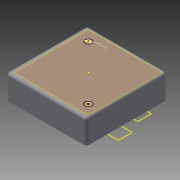
# Autodesk Inventor part: enclosure2
Saved by Autodesk Inventor 2013 (Build 170138000, 138)
## iProperties
Created: 2013-01-07
Part Number: enclosure2
Material: Generic
Document SubType Name: Modeling
Designer: md
Density: 1 g/cm^3
Author: md
Autodesk Inventor part; units mm, degrees
ref_plane "YZ Plane" through (0, 0, 0) normal (1, 0, 0) x (0, 1, 0)
ref_plane "XZ Plane" through (0, 0, 0) normal (0, 1, 0) x (-1, 0, 0)
ref_plane "XY Plane" through (0, 0, 0) normal (0, 0, 1) x (1, 0, 0)
derived "PCB-Model.ipt"
sketch "Platine" plane through (0, 0, 0) normal (0, 0, 1) x (1, 0, 0)
  line L0 (-25, -25) -> (25, -25)
  line L1 (25, -25) -> (25, 25)
  line L2 (25, 25) -> (-25, 25)
  line L3 (-25, 25) -> (-25, -25)
  line L4 (-25, -25) -> (25, 25)
  line L5 (25, -25) -> (-25, 25)
  line L6 (-30.8, -10.2) -> (-8.8, -10.2)
  line L7 (-8.8, -10.2) -> (-8.8, 5.8)
  line L8 (-8.8, 5.8) -> (-30.8, 5.8)
  line L9 (-30.8, 5.8) -> (-30.8, -10.2)
  line L10 (33.4, -11.2) -> (19.4, -11.2)
  line L11 (19.4, -11.2) -> (19.4, -1.04)
  line L12 (19.4, -1.04) -> (33.4, -1.04)
  line L13 (33.4, -1.04) -> (33.4, -11.2)
  line L14 (14.5, 8) -> (28.5, 8)
  line L15 (28.5, 8) -> (28.5, 18)
  line L16 (28.5, 18) -> (14.5, 18)
  line L17 (14.5, 18) -> (14.5, 8)
  circle A0 centre (-20, 20) radius 1.5
  circle A1 centre (20, -20) radius 1.5
  point P0 (0, 0)
  point P1 (0, 0)
derived "enclosure1.ipt"
sketch "Aussenmass" plane through (-25, 25, -9) normal (0, 0, 1) x (1, 0, 0)
  line L0 (-5.8, 5) -> (53.5, 5)
  line L1 (53.5, 5) -> (53.5, -55)
  line L2 (53.5, -55) -> (-5.8, -55)
  line L3 (-5.8, -55) -> (-5.8, 5)
  line L4 (-5.8, -19.2) -> (-5.8, -35.2)
  line L5 (53.5, -17) -> (53.5, -7)
  point P0 (25, -25)
ref_plane "Bottom of Case_1" through (-25, 25, -9) normal (0, 0, 1) x (1, 0, 0)
ref_plane "Work Plane4" through (-25, 25, 21) normal (0, 0, 1) x (1, 0, 0)
sketch "Sketch4" plane through (-25, 25, 21) normal (0, 0, 1) x (1, 0, 0)
  line L0 (-5.7866, 4.9846) -> (53.5589, 4.9846)
  line L1 (53.5589, 4.9846) -> (53.5589, -54.9846)
  line L2 (53.5589, -54.9846) -> (-5.7866, -54.9846)
  line L3 (-5.7866, -54.9846) -> (-5.7866, 4.9846)
  point P0 (25, -25)
  constraints: 8 end point, 2 parallel, 1 horizontal, 1 perpendicular
extrude "Extrusion1" add sketch "Sketch4" against normal blind 18
fillet "Fillet1" radius 2 7 edges at (-30.7866, -29.9846, 12) (-1.1138, -29.9846, 21) (-30.7866, 0, 21) (28.5589, 29.9846, 12) (28.5589, 0, 21) (28.5589, -29.9846, 12) (-30.7866, 29.9846, 12)
fillet "Fillet2" radius 2 3 edges at (-1.1138, 29.9846, 21) (27.9731, 29.3988, 20.4142) (-30.2008, 29.3988, 20.4142)
shell "Shell2" thickness 2 removed faces 1 at (-11.0048, -9.3282, 3)
sketch "Lochpositionen" plane through (-25, 25, 21) normal (0, 0, 1) x (1, 0, 0)
  circle A0 centre (5, -5) radius 1.5 projected
  circle A1 centre (45, -45) radius 1.5 projected
  circle A2 centre (5, -5) radius 2.5
  circle A3 centre (45, -45) radius 2.5
  point P0 (25, -25)
  dimension "d19" = 5
  constraints: 2 centre point, 2 coincident, 1 equal radius
  measures "d19" diameter of A2
extrude "Extrusion2" add sketch "Lochpositionen" against normal blind 18
hole "Hole2" at (-20, 20, 21) direction (0, 0, -1) diameter 3 end through all countersink diameter 4 countersink angle 90
hole "Hole3" at (20, -20, 21) direction (0, 0, -1) diameter 3 end through all countersink diameter 4 countersink angle 90
fillet "Fillet3" radius 3 2 edges at (17.5, -20, 19) (-22.5, 20, 19)
body "Solid1"
